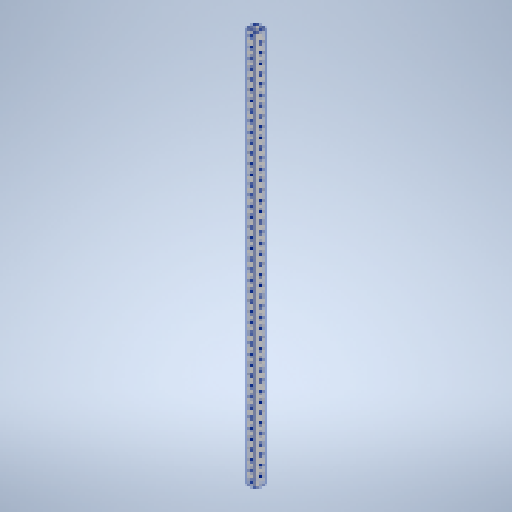
# Autodesk Inventor part: 10x10x431
Saved by Autodesk Inventor 2025 (Build 290162000, 162)
## iProperties
Created: 2025-03-04
Part Number: 10x10x431
Material: アルミニウム 6061
Document SubType Name: Modeling
Designer: Zhopa
Density: 2.7 g/cm^3
Appearance: アルミニウム - フラット
Mass: 38.6487 g
Surface Area: 303.029 cm^2
Volume: 14.3143 cm^3
Author: Zhopa
Autodesk Inventor part; units mm, degrees
ref_plane "YZ Plane" through (0, 0, 0) normal (1, 0, 0) x (0, 1, 0)
ref_plane "XZ Plane" through (0, 0, 0) normal (0, 1, 0) x (-1, 0, 0)
ref_plane "XY Plane" through (0, 0, 0) normal (0, 0, 1) x (1, 0, 0)
sketch "Sketch1" plane through (0, 0, 0) normal (0, 1, 0) x (-1, 0, 0)
  line L0 (5, 5) -> (-5, 5)
  line L1 (-5, 5) -> (-5, -5)
  line L2 (-5, -5) -> (5, -5)
  line L3 (5, -5) -> (5, 5)
  line L4 (5, 5) -> (-5, -5) construction
  line L5 (-5, 5) -> (5, -5) construction
  line L6 (4, 4) -> (-4, 4)
  line L7 (-4, 4) -> (-4, -4)
  line L8 (-4, -4) -> (4, -4)
  line L9 (4, -4) -> (4, 4)
  line L10 (4, 4) -> (-4, -4) construction
  line L11 (-4, 4) -> (4, -4) construction
  point P0 (0, 0)
  dimension "d0" = 10
  dimension "d1" = 10
  dimension "d2" = 8
  dimension "d3" = 8
  constraints: 24 end point, 4 midpoint, 4 parallel, 2 horizontal, 2 perpendicular
  measures "d0" distance of L2.end L1.end
  measures "d1" distance of L1.end L0.end
  measures "d2" distance of L8.end L7.end
  measures "d3" distance of L7.end L6.end
extrude "Extrusion1" add sketch "Sketch1" along normal blind 431
sketch "Sketch2" plane through (-5, 0, 5) normal (0, 0, 1) x (1, 0, 0)
  line L0 (0, 0) -> (10, 0) projected
  line L1 (0, 0) -> (0, 431) projected
  line L2 (0, 0) -> (0, 8.9832)
  point P0 (5, 0)
  point P1 (5, 5)
  point P2 (5, 15)
  point P3 (5, 15)
  point P4 (5, 25)
  point P5 (5, 25)
  point P6 (5, 35)
  point P7 (5, 35)
  point P8 (5, 45)
  point P9 (5, 45)
  point P10 (5, 55)
  point P11 (5, 55)
  point P12 (5, 65)
  point P13 (5, 65)
  point P14 (5, 75)
  point P15 (5, 75)
  point P16 (5, 85)
  point P17 (5, 85)
  point P18 (5, 95)
  point P19 (5, 95)
  point P20 (5, 105)
  point P21 (5, 105)
  point P22 (5, 115)
  point P23 (5, 115)
  point P24 (5, 125)
  point P25 (5, 125)
  point P26 (5, 135)
  point P27 (5, 135)
  point P28 (5, 145)
  point P29 (5, 145)
  point P30 (5, 155)
  point P31 (5, 155)
  point P32 (5, 165)
  point P33 (5, 165)
  point P34 (5, 175)
  point P35 (5, 175)
  point P36 (5, 185)
  point P37 (5, 185)
  point P38 (5, 195)
  point P39 (5, 195)
  point P40 (5, 205)
  point P41 (5, 205)
  point P42 (5, 215)
  point P43 (5, 215)
  point P44 (5, 225)
  point P45 (5, 225)
  point P46 (5, 235)
  point P47 (5, 235)
  point P48 (5, 245)
  point P49 (5, 245)
  point P50 (5, 255)
  point P51 (5, 255)
  point P52 (5, 265)
  point P53 (5, 265)
  point P54 (5, 275)
  point P55 (5, 275)
  point P56 (5, 285)
  point P57 (5, 285)
  point P58 (5, 295)
  point P59 (5, 295)
  point P60 (5, 305)
  point P61 (5, 305)
  point P62 (5, 315)
  point P63 (5, 315)
  point P64 (5, 325)
  point P65 (5, 325)
  point P66 (5, 335)
  point P67 (5, 335)
  point P68 (5, 345)
  point P69 (5, 345)
  point P70 (5, 355)
  point P71 (5, 355)
  point P72 (5, 365)
  point P73 (5, 365)
  point P74 (5, 375)
  point P75 (5, 375)
  point P76 (5, 385)
  point P77 (5, 385)
  point P78 (5, 395)
  point P79 (5, 395)
  point P80 (5, 405)
  point P81 (5, 405)
  point P82 (5, 415)
  point P83 (5, 415)
  point P84 (5, 425)
  point P85 (5, 425)
  point P86 (5, 435)
  point P87 (5, 426)
  dimension "d6" = 5
  dimension "d7" = 10
  dimension "d10" = 10
  dimension "d38" = 1
  constraints: 2 end point, 1 point on line, 1 vertical, 84 other
  measures "d6" distance from line of L0 point (5, 5)
  measures "d7" distance of point (5, 5) point (5, 15)
  measures "d10" distance of point (5, 5) point (5, 15)
  measures "d38" distance of point (5, 425) point (5, 426)
hole "Hole1" at (0, 5, 5) at (0, 15, 5) at (0, 25, 5) at (0, 35, 5) at (0, 45, 5) at (0, 55, 5) at (0, 65, 5) at (0, 75, 5) at (0, 85, 5) at (0, 95, 5) at (0, 105, 5) at (0, 115, 5) at (0, 125, 5) at (0, 135, 5) at (0, 145, 5) at (0, 155, 5) at (0, 165, 5) at (0, 175, 5) at (0, 185, 5) at (0, 195, 5) at (0, 205, 5) at (0, 215, 5) at (0, 225, 5) at (0, 235, 5) at (0, 245, 5) at (0, 255, 5) at (0, 265, 5) at (0, 275, 5) at (0, 285, 5) at (0, 295, 5) at (0, 305, 5) at (0, 315, 5) at (0, 325, 5) at (0, 335, 5) at (0, 345, 5) at (0, 355, 5) at (0, 365, 5) at (0, 375, 5) at (0, 385, 5) at (0, 395, 5) at (0, 405, 5) at (0, 415, 5) at (0, 435, 5) at (0, 426, 5) direction (0, 0, -1) diameter 3 depth 80.45
sketch "Sketch3" plane through (5, 0, 5) normal (1, 0, 0) x (0, 0, -1)
  line L0 (0, 0) -> (10, 0) projected
  line L1 (0, 0) -> (0, 431) projected
  line L2 (0, 0) -> (0, 6.3724)
  point P0 (5, 0)
  point P1 (5, 10)
  point P2 (5, 20)
  point P3 (5, 20)
  point P4 (5, 30)
  point P5 (5, 30)
  point P6 (5, 40)
  point P7 (5, 40)
  point P8 (5, 50)
  point P9 (5, 50)
  point P10 (5, 60)
  point P11 (5, 60)
  point P12 (5, 70)
  point P13 (5, 70)
  point P14 (5, 80)
  point P15 (5, 80)
  point P16 (5, 90)
  point P17 (5, 90)
  point P18 (5, 100)
  point P19 (5, 100)
  point P20 (5, 110)
  point P21 (5, 110)
  point P22 (5, 120)
  point P23 (5, 120)
  point P24 (5, 130)
  point P25 (5, 130)
  point P26 (5, 140)
  point P27 (5, 140)
  point P28 (5, 150)
  point P29 (5, 150)
  point P30 (5, 160)
  point P31 (5, 160)
  point P32 (5, 170)
  point P33 (5, 170)
  point P34 (5, 180)
  point P35 (5, 180)
  point P36 (5, 190)
  point P37 (5, 190)
  point P38 (5, 200)
  point P39 (5, 200)
  point P40 (5, 210)
  point P41 (5, 210)
  point P42 (5, 220)
  point P43 (5, 220)
  point P44 (5, 230)
  point P45 (5, 230)
  point P46 (5, 240)
  point P47 (5, 240)
  point P48 (5, 250)
  point P49 (5, 250)
  point P50 (5, 260)
  point P51 (5, 260)
  point P52 (5, 270)
  point P53 (5, 270)
  point P54 (5, 280)
  point P55 (5, 280)
  point P56 (5, 290)
  point P57 (5, 290)
  point P58 (5, 300)
  point P59 (5, 300)
  point P60 (5, 310)
  point P61 (5, 310)
  point P62 (5, 320)
  point P63 (5, 320)
  point P64 (5, 330)
  point P65 (5, 330)
  point P66 (5, 340)
  point P67 (5, 340)
  point P68 (5, 350)
  point P69 (5, 350)
  point P70 (5, 360)
  point P71 (5, 360)
  point P72 (5, 370)
  point P73 (5, 370)
  point P74 (5, 380)
  point P75 (5, 380)
  point P76 (5, 390)
  point P77 (5, 390)
  point P78 (5, 400)
  point P79 (5, 400)
  point P80 (5, 410)
  point P81 (5, 410)
  point P82 (5, 420)
  point P83 (5, 420)
  point P84 (5, 430)
  point P85 (5, 430)
  point P86 (5, 440)
  dimension "d22" = 10
  dimension "d23" = 10
  dimension "d26" = 10
  constraints: 2 end point, 1 point on line, 1 vertical, 84 other
  measures "d22" distance from line of point (5, 10) L0
  measures "d23" distance of point (5, 10) point (5, 20)
  measures "d26" distance of point (5, 10) point (5, 20)
hole "Hole2" at (5, 10, 0) at (5, 20, 0) at (5, 30, 0) at (5, 40, 0) at (5, 50, 0) at (5, 60, 0) at (5, 70, 0) at (5, 80, 0) at (5, 90, 0) at (5, 100, 0) at (5, 110, 0) at (5, 120, 0) at (5, 130, 0) at (5, 140, 0) at (5, 150, 0) at (5, 160, 0) at (5, 170, 0) at (5, 180, 0) at (5, 190, 0) at (5, 200, 0) at (5, 210, 0) at (5, 220, 0) at (5, 230, 0) at (5, 240, 0) at (5, 250, 0) at (5, 260, 0) at (5, 270, 0) at (5, 280, 0) at (5, 290, 0) at (5, 300, 0) at (5, 310, 0) at (5, 320, 0) at (5, 330, 0) at (5, 340, 0) at (5, 350, 0) at (5, 360, 0) at (5, 370, 0) at (5, 380, 0) at (5, 390, 0) at (5, 400, 0) at (5, 410, 0) at (5, 420, 0) at (5, 440, 0) direction (-1, 0, 0) diameter 3 depth 80.45
body "Solid1"
